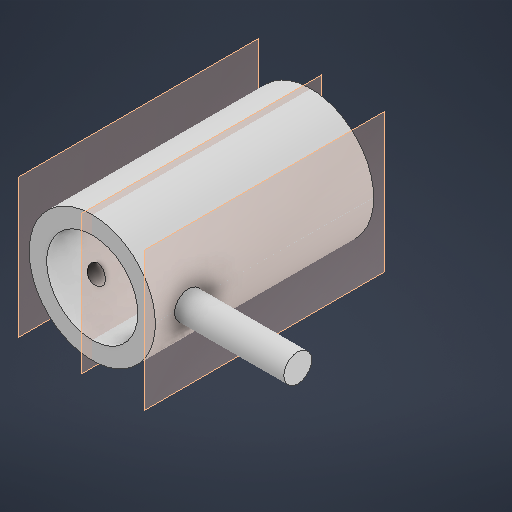
# Autodesk Inventor part: Swivel Part
Saved by Autodesk Inventor 2026.2 (Build 302298000, 298)
## iProperties
Created: 2026-02-07
Part Number: Swivel Part
Material: Generic
Document SubType Name: Modeling
Designer: chigg
Density: 1 g/cm^3
Appearance: Default
Author: chigg
Autodesk Inventor part; units mm, degrees
ref_plane "XZ Plane" through (0, 0, 0) normal (0, 1, 0) x (-1, 0, 0)
ref_plane "XY Plane" through (0, 0, 0) normal (0, 0, 1) x (1, 0, 0)
sketch "Sketch1" plane through (0, 0, 0) normal (0, 0, 1) x (1, 0, 0)
  circle A0 centre (0, 0) radius 7.3435
  constraints: 1 centre point, 1 coincident
extrude "Extrusion1" add sketch "Sketch1" along normal blind 25.4
sketch "Sketch2" plane through (0, 0, 25.4) normal (0, 0, 1) x (1, 0, 0)
  circle A0 centre (0, 0) radius 5.2916
  constraints: 1 centre point, 1 coincident
extrude "Extrusion2" cut sketch "Sketch2" against normal blind 20.32
sketch "Sketch3" plane through (0, 0, 0) normal (0, 0, -1) x (-1, 0, 0)
  circle A0 centre (0, 0) radius 0.3929
  constraints: 1 centre point, 1 coincident
extrude "Extrusion3" cut sketch "Sketch3" against normal through all
ref_plane "Work Plane1" through (7.3406, 0, 0) normal (1, 0, 0) x (0, 1, 0)
sketch "Sketch6" plane through (7.3406, 0, 0) normal (1, 0, 0) x (0, 1, 0)
  circle A0 centre (0, 21.5391) radius 1.6203
  point P0 (0, 0)
  constraints: 1 centre point
extrude "Extrusion4" add sketch "Sketch6" along normal blind 12.7
ref_plane "Work Plane2" through (-7.3406, 0, 0) normal (1, 0, 0) x (0, 1, 0)
sketch "Sketch7" plane through (-7.3406, 0, 0) normal (1, 0, 0) x (0, 1, 0)
  circle A0 centre (-3.11, 20.6976) radius 0.8484
  circle A1 centre (2.4665, 20.6976) radius 0.8501
  point P0 (0, 0)
  constraints: 2 centre point
extrude "Extrusion5" cut sketch "Sketch7" along normal blind 3.81
body "Solid1"
